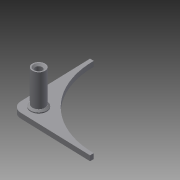
# Autodesk Inventor part: Speaker Nuts
Saved by Autodesk Inventor 2014 SP2 (Build 180246200, 246)
## iProperties
Created: 2015-08-11
Part Number: Speaker Nuts
Material: Generic
Document SubType Name: Modeling
Designer: Devon
Density: 1 g/cm^3
Appearance: Default
Author: Devon
Autodesk Inventor part; units mm, degrees
ref_plane "YZ Plane" through (0, 0, 0) normal (1, 0, 0) x (0, 1, 0)
ref_plane "XZ Plane" through (0, 0, 0) normal (0, 1, 0) x (-1, 0, 0)
ref_plane "XY Plane" through (0, 0, 0) normal (0, 0, 1) x (1, 0, 0)
sketch "Sketch1" plane through (0, 0, 0) normal (0, 1, 0) x (-1, 0, 0)
  arc A0 (25.019, 0) -> (0, 25.019) centre (0, 0) ccw
  line L0 (26.2128, 0) -> (25.4953, 22.4234)
  line L1 (22.4234, 25.4953) -> (0, 26.2128)
  arc A1 (25.4953, 22.4234) -> (22.4234, 25.4953) centre (22.3219, 22.3219) ccw
  line L2 (26.2128, 0) -> (25.019, 0)
  line L3 (0, 26.2128) -> (0, 25.019)
  point P0 (25.4, 25.4)
  point P1 (25.4, -25.4)
  dimension "d0" = 50.038
  dimension "d3" = 50.8
  dimension "d9" = 3.175
  constraints: 8 end point, 4 point on circle, 2 centre point, 2 point on line, 2 tangent, 1 coincident, 1 horizontal, 1 perpendicular
  measures "d0" diameter of A0
  measures "d3" distance of point (25.4, 25.4) point (25.4, -25.4)
  measures "d9" radius of A1
extrude "Extrusion1" add sketch "Sketch1" along normal blind 1.5875
sketch "Sketch2" plane through (0, 1.5875, 0) normal (0, 1, 0) x (1, 0, 0)
  circle A0 centre (-21.129, -21.129) radius 1.9812
  circle A1 centre (-21.129, -21.129) radius 1.0795
  dimension "d12" = 3.9624
  dimension "d13" = 2.159
  constraints: 2 centre point, 1 coincident
  measures "d12" diameter of A0
  measures "d13" diameter of A1
extrude "Extrusion2" add sketch "Sketch2" along normal blind 10.795
sketch "Sketch3" plane through (0, 1.5875, 0) normal (0, 1, 0) x (1, 0, 0)
  circle A0 centre (-21.129, -21.129) radius 1.9812 projected
  circle A1 centre (-21.129, -21.129) radius 2.54
  dimension "d16" = 5.08
  constraints: 1 centre point, 1 coincident
  measures "d16" diameter of A1
extrude "Extrusion3" add sketch "Sketch3" along normal blind 0.7937
chamfer "Chamfer1" distance 0.508 angle 45 1 edges at (-23.669, 2.3812, 21.129)
chamfer "Chamfer2" distance 0.508 angle 45 1 edges at (-22.2085, 12.3825, 21.129)
body "Solid1"
